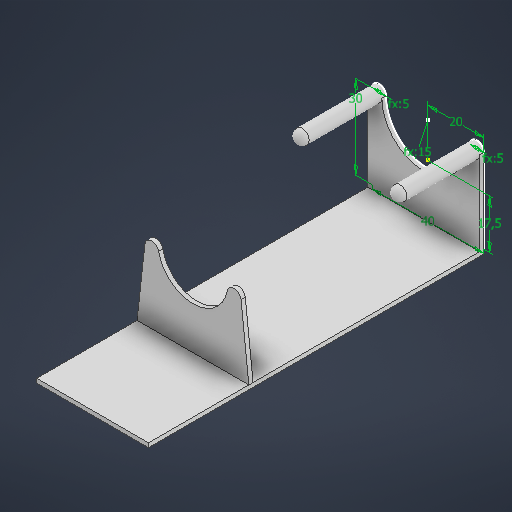
# Autodesk Inventor part: my_portafilter_holder_23ipt
Saved by Autodesk Inventor 2026 (Build 300175000, 175)
## iProperties
Created: 2025-04-17
Part Number: my_portafilter_holder_23ipt
Material: Generic
Document SubType Name: Modeling
Designer: Paul Juschitz
Density: 1 g/cm^3
Appearance: Default
Author: Paul Juschitz
Autodesk Inventor part; units mm, degrees
ref_plane "YZ Plane" through (0, 0, 0) normal (1, 0, 0) x (0, 1, 0)
ref_plane "XZ Plane" through (0, 0, 0) normal (0, 1, 0) x (-1, 0, 0)
ref_plane "XY Plane" through (0, 0, 0) normal (0, 0, 1) x (1, 0, 0)
sketch "Sketch1" plane through (0, 0, 0) normal (0, 0, 1) x (1, 0, 0)
  line L0 (20, 12.5) -> (20, -17.5)
  line L1 (20, -17.5) -> (-20, -17.5)
  line L2 (-20, -17.5) -> (-20, 12.5)
  circle A0 centre (-17.5, 12.5) radius 2.5
  circle A1 centre (17.5, 12.5) radius 2.5
  arc A2 (-15, 12.5) -> (15, 12.5) centre (0, 12.5) ccw
  point P0 (0, 0)
  dimension "d0" = 40
  dimension "d2" = 5
  dimension "d3" = 5
  dimension "d4" = 30
  dimension "d5" = 20
  dimension "d6" = 17.5
  dimension "d7" = 15
  constraints: 6 end point, 6 point on circle, 4 tangent, 3 centre point, 1 horizontal, 1 horizontal alignment, 1 parallel, 1 perpendicular
  measures "d0" distance of L0.end L1.end
  measures "d2" diameter of A0
  measures "d3" diameter of A1
  measures "d4" distance of L1.end L2.end
  measures "d5" distance from line of point (0, 0) L0
  measures "d6" distance from line of point (0, 0) L1
  measures "d7" radius of A2
extrude "Extrusion1" add sketch "Sketch1" along normal blind 1.5 contours L0 L1 L2 A0 A2 A1
extrude "Extrusion2" add sketch "Sketch1" along normal blind 30 contours A1 | A0
fillet "Fillet1" radius 2.5 2 edges at (-20, 12.5, 30) (15, 12.5, 30)
sketch "Sketch2" plane through (0, 0, 0) normal (0, 0, 1) x (1, 0, 0)
  line L0 (-20, -17.5) -> (20, -17.5) projected
  line L1 (-20, -17.5) -> (20, -17.5) projected
  line L2 (-20, -17.5) -> (20, -17.5)
  line L3 (20, -17.5) -> (20, -19)
  line L4 (20, -19) -> (-20, -19)
  line L5 (-20, -19) -> (-20, -17.5)
  point P0 (0, 0)
  dimension "d13" = 1.5
  constraints: 8 end point, 3 perpendicular, 1 collinear
  measures "d13" distance of L4.end L0.start
extrude "Extrusion3" add sketch "Sketch2" along normal blind 120
sketch "Sketch5" plane through (-20, -17.5, 1.5) normal (0, 1, 0) x (1, 0, 0)
  line L0 (0, 0) -> (0, -118.5) projected
  line L1 (40, 0) -> (40, -118.5) projected
  line L2 (0, -81.0917) -> (40, -81.0917)
  line L3 (40, -81.0917) -> (40, -82.5917)
  line L4 (40, -82.5917) -> (0, -82.5917)
  line L5 (0, -82.5917) -> (0, -81.0917)
  line L6 (0, 0) -> (40, 0) projected
  point P0 (20, 1.5)
  point P1 (0, -82.5917)
  dimension "d25" = 1.5
  dimension "d26" = 81.0917
  constraints: 8 end point, 2 parallel, 2 point on line, 1 horizontal, 1 perpendicular
  measures "d25" distance between parallel lines of L4 L2
  measures "d26" distance between parallel lines of L6 L2
extrude "Extrusion5" add sketch "Sketch5" along normal blind 30 contours L2 L1 L4 L0
sketch "Sketch6" plane through (-20, -17.5, 84.0917) normal (0, 0, 1) x (1, 0, 0)
  line L0 (0, 30) -> (0, -1.5) projected
  line L1 (0, -0.0564) -> (0, 30)
  line L2 (40, 30) -> (0, 30) projected
  line L3 (0, 30) -> (40, 30)
  line L4 (40, 30) -> (40, -0.0564)
  line L5 (40, -0.0564) -> (0, -0.0564)
  line L6 (0, -0.0564) -> (2.7921, 25.0554)
  arc A0 (7.7306, 25.2572) -> (2.7921, 25.0554) centre (5.2768, 24.7792) ccw
  arc A1 (7.7306, 25.2572) -> (32.2694, 25.2572) centre (20, 27.6473) ccw
  arc A2 (37.2079, 25.0554) -> (32.2694, 25.2572) centre (34.7232, 24.7792) ccw
  line L7 (37.2079, 25.0554) -> (40, -0.0564)
  line L8 (20, -0.0564) -> (20, 30)
  point P0 (20, 17.5)
  dimension "d29" = 2.5
  dimension "d30" = 12.5
  dimension "d31" = 29.4465
  dimension "d32" = 6.344
  dimension "d33" = 30.0564
  constraints: 14 end point, 6 point on circle, 4 tangent, 3 centre point, 2 collinear, 2 midpoint, 2 perpendicular, 1 equal radius, 1 horizontal alignment, 1 point on line, 1 other
  measures "d29" radius of A0
  measures "d30" radius of A1
  measures "d31" distance of A2.centre A0.centre
  measures "d32" angle of L0 L7
  measures "d33" distance between parallel lines of L5 L2
extrude "Extrusion6" cut sketch "Sketch6" against normal up to surface (1.5 mm away) contours L2 L8 A1 A0 L6 L0 | L2 L4 L7 A2 A1 L8
equation "\"d2\" = arm_thickness"
equation "\"d3\" = arm_thickness"
equation "\"d7\" = 3 * arm_thickness"
equation "\"d8\" = material_thickness"
equation "\"d10\" = arm_length"
equation "\"d12\" = 0.5 * arm_thickness"
equation "\"d13\" = material_thickness"
equation "\"d25\" = material_thickness"
equation "\"d29\" = 0.5 * arm_thickness"
equation "\"arm_thickness\" = 5"
equation "\"material_thickness\" = 1.5"
equation "\"arm_length\" = 30"
body "Solid1"
